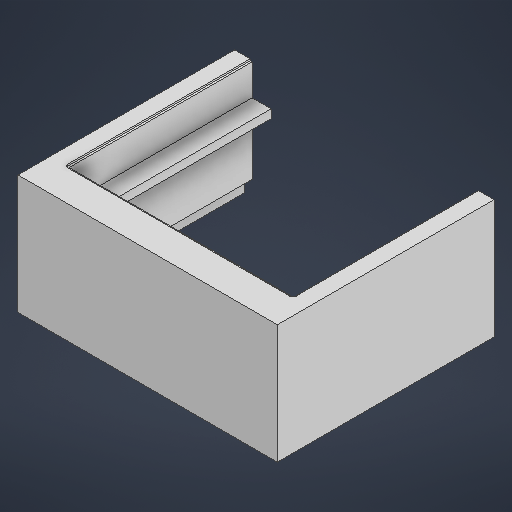
# Autodesk Inventor part: Enclosure
Saved by Autodesk Inventor 2025.2 (Build 292293000, 293)
## iProperties
Created: 2025-02-10
Part Number: Enclosure
Material: Generic
Document SubType Name: Modeling
Designer: elier
Density: 1 g/cm^3
Appearance: Default
Author: elier
Autodesk Inventor part; units mm, degrees
ref_plane "YZ Plane" through (0, 0, 0) normal (1, 0, 0) x (0, 1, 0)
ref_plane "XZ Plane" through (0, 0, 0) normal (0, 1, 0) x (-1, 0, 0)
ref_plane "XY Plane" through (0, 0, 0) normal (0, 0, 1) x (1, 0, 0)
sketch "Sketch1" plane through (0, 0, 0) normal (0, 1, 0) x (-1, 0, 0)
  line L0 (-83.5, 139.5) -> (83.5, 139.5)
  line L1 (83.5, 139.5) -> (83.5, -139.5)
  line L2 (83.5, -139.5) -> (-83.5, -139.5)
  line L3 (-83.5, -139.5) -> (-83.5, 139.5)
  line L4 (-83.5, 139.5) -> (83.5, -139.5) construction
  line L5 (83.5, 139.5) -> (-83.5, -139.5) construction
  point P0 (0, 0)
  dimension "d0" = 167
  dimension "d1" = 279
  constraints: 12 end point, 2 midpoint, 2 parallel, 1 horizontal, 1 perpendicular
  measures "d0" distance of L1.end L2.end
  measures "d1" distance of L0.end L1.end
extrude "Extrusion1" add sketch "Sketch1" along normal blind 26.6
sketch "Sketch2" plane through (0, 26.6, 0) normal (0, 1, 0) x (1, 0, 0)
  line L0 (71.5, -119.5) -> (-71.5, -119.5)
  line L1 (-73.5, -117.5) -> (-73.5, 117.5)
  line L2 (-71.5, 119.5) -> (71.5, 119.5)
  line L3 (73.5, 117.5) -> (73.5, -117.5)
  line L4 (73.5, -119.5) -> (-73.5, 119.5) construction
  line L5 (-73.5, -119.5) -> (73.5, 119.5) construction
  arc A0 (-73.5, -117.5) -> (-71.5, -119.5) centre (-71.5, -117.5) ccw
  arc A1 (-71.5, 119.5) -> (-73.5, 117.5) centre (-71.5, 117.5) ccw
  arc A2 (73.5, 117.5) -> (71.5, 119.5) centre (71.5, 117.5) ccw
  arc A3 (71.5, -119.5) -> (73.5, -117.5) centre (71.5, -117.5) ccw
  point P0 (0, 0)
  dimension "d4" = 147
  dimension "d5" = 239
  dimension "d6" = 2
  constraints: 12 end point, 8 point on circle, 8 point on line, 8 tangent, 4 centre point, 3 equal radius, 2 midpoint, 2 parallel, 1 horizontal, 1 perpendicular
  measures "d4" distance of L4.end L5.end
  measures "d5" distance of L5.start L4.end
  measures "d6" radius of A0
extrude "Extrusion2" cut sketch "Sketch2" against normal blind 1.1
sketch "Sketch3" plane through (0, 25.5, 0) normal (0, 1, 0) x (1, 0, 0)
  line L0 (-73.5, -117.5) -> (-73.5, 117.5) projected
  line L1 (71.5, -119.5) -> (-71.5, -119.5) projected
  line L2 (-72.25, -117.83) -> (72.25, -117.83)
  line L3 (72.25, -117.83) -> (72.25, 112.27)
  line L4 (72.25, 112.27) -> (-72.25, 112.27)
  line L5 (-72.25, 112.27) -> (-72.25, -117.83)
  point P0 (0, 0)
  dimension "d9" = 1.25
  dimension "d10" = 1.67
  dimension "d11" = 144.5
  dimension "d12" = 230.1
  constraints: 8 end point, 2 parallel, 1 horizontal, 1 perpendicular
  measures "d9" distance from line of L0 L2.start
  measures "d10" distance from line of L1 L2.start
  measures "d11" distance of L4.end L3.end
  measures "d12" distance of L3.end L2.end
extrude "Extrusion3" cut sketch "Sketch3" against normal blind 20
sketch "Sketch4" plane through (0, 5.5, 0) normal (0, 1, 0) x (1, 0, 0)
  circle A0 centre (-66.5, -111.83) radius 2
  line L0 (72.25, -117.83) -> (-72.25, -117.83) projected
  line L1 (-72.25, -117.83) -> (-72.25, 112.27) projected
  circle A1 centre (66.5, -111.83) radius 2
  line L2 (72.25, 112.27) -> (72.25, -117.83) projected
  circle A2 centre (-66.5, 106.27) radius 2
  line L3 (-72.25, 112.27) -> (72.25, 112.27) projected
  circle A3 centre (66.5, 106.27) radius 2
  point P0 (0, 0)
  dimension "d15" = 4
  dimension "d16" = 6
  dimension "d17" = 5.75
  dimension "d18" = 4
  dimension "d19" = 6
  dimension "d20" = 5.75
  dimension "d21" = 4
  dimension "d22" = 5.75
  dimension "d23" = 6
  dimension "d24" = 4
  dimension "d25" = 6
  dimension "d26" = 5.75
  constraints: 4 centre point
  measures "d15" diameter of A0
  measures "d16" distance from line of L0 A0.centre
  measures "d17" distance from line of L1 A0.centre
  measures "d18" diameter of A1
  measures "d19" distance from line of L0 A1.centre
  measures "d20" distance from line of L2 A1.centre
  measures "d21" diameter of A2
  measures "d22" distance from line of L1 A2.centre
  measures "d23" distance from line of L3 A2.centre
  measures "d24" diameter of A3
  measures "d25" distance from line of L3 A3.centre
  measures "d26" distance from line of L2 A3.centre
extrude "Extrusion4" add sketch "Sketch4" along normal blind 10.3 contours A0 | A1 | A2 | A3
sketch "Sketch5" plane through (0, 5.5, 0) normal (0, 1, 0) x (1, 0, 0)
  circle A0 centre (-66.5, -111.83) radius 2 projected
  circle A1 centre (-66.5, -111.83) radius 1.25
  circle A2 centre (-66.5, 106.27) radius 2 projected
  circle A3 centre (-66.5, 106.27) radius 1.25
  circle A4 centre (66.5, 106.27) radius 2 projected
  circle A5 centre (66.5, 106.27) radius 1.25
  circle A6 centre (66.5, -111.83) radius 1.25
  point P0 (0, 0)
  dimension "d29" = 2.5
  dimension "d30" = 2.5
  dimension "d31" = 2.5
  dimension "d32" = 2.5
  constraints: 4 centre point, 3 coincident
  measures "d29" diameter of A1
  measures "d30" diameter of A3
  measures "d31" diameter of A5
  measures "d32" diameter of A6
extrude "Extrusion5" cut sketch "Sketch5" along normal blind 10.3 and the other way blind 5.5 contours A1 | A3 | A5 | A6
sketch "Sketch8" plane through (0, 0, 0) normal (0, -1, 0) x (1, 0, 0)
  circle A0 centre (66.5, 111.83) radius 1.25 projected
  circle A1 centre (66.5, 111.83) radius 1.75
  circle A2 centre (66.5, -106.27) radius 1.25 projected
  circle A3 centre (66.5, -106.27) radius 1.75
  circle A4 centre (-66.5, -106.27) radius 1.25 projected
  circle A5 centre (-66.5, -106.27) radius 1.75
  circle A6 centre (-66.5, 111.83) radius 1.75
  point P0 (0, 0)
  dimension "d49" = 3.5
  dimension "d50" = 3.5
  dimension "d51" = 3.5
  dimension "d52" = 3.5
  constraints: 4 centre point, 3 coincident
  measures "d49" diameter of A1
  measures "d50" diameter of A3
  measures "d51" diameter of A5
  measures "d52" diameter of A6
extrude "Extrusion8" cut sketch "Sketch8" against normal blind 13.8
sketch "Sketch9" plane through (0, 5.5, 0) normal (0, 1, 0) x (1, 0, 0)
  line L0 (60, -100) -> (-60, -100)
  line L1 (-60, -100) -> (-60, 100)
  line L2 (-60, 100) -> (60, 100)
  line L3 (60, 100) -> (60, -100)
  line L4 (60, -100) -> (-60, 100) construction
  line L5 (-60, -100) -> (60, 100) construction
  point P0 (0, 0)
  dimension "d55" = 120
  dimension "d56" = 200
  constraints: 12 end point, 2 midpoint, 2 parallel, 1 horizontal, 1 perpendicular
  measures "d55" distance of L1.end L2.end
  measures "d56" distance of L0.end L1.end
extrude "Extrusion9" cut sketch "Sketch9" against normal blind 5.8
sketch "Sketch10" plane through (0, 0, 0) normal (0, -1, 0) x (1, 0, 0)
  line L0 (83.5, 139.5) -> (83.5, -139.5) projected
  line L1 (-83.5, -139.5) -> (-83.5, 139.5) projected
  line L2 (83.5, 139.5) -> (-83.5, 139.5)
  line L3 (-83.5, 139.5) -> (-83.5, -139.5)
  line L4 (-83.5, -139.5) -> (83.5, -139.5)
  line L5 (83.5, -139.5) -> (83.5, 139.5)
  line L6 (72.25, -115.05) -> (-72.25, -115.05)
  line L7 (-72.25, -115.05) -> (-72.25, 115.05)
  line L8 (-72.25, 115.05) -> (72.25, 115.05)
  line L9 (72.25, 115.05) -> (72.25, -115.05)
  line L10 (72.25, -115.05) -> (-72.25, 115.05) construction
  line L11 (-72.25, -115.05) -> (72.25, 115.05) construction
  line L12 (-83.5, -139.5) -> (83.5, -139.5)
  line L13 (83.5, -139.5) -> (83.5, 139.5)
  line L14 (83.5, 139.5) -> (-83.5, 139.5)
  line L15 (-83.5, 139.5) -> (-83.5, -139.5)
  point P0 (0, 0)
  point P1 (71.5, 119.5)
  dimension "d67" = 144.5
  dimension "d68" = 230.1
  constraints: 28 end point, 6 parallel, 3 horizontal, 3 perpendicular, 2 midpoint
  measures "d67" distance of L7.end L8.end
  measures "d68" distance of L6.end L7.end
extrude "Extrusion10" add sketch "Sketch10" along normal blind 40
sketch "Sketch12" plane through (0, -40, 0) normal (0, -1, 0) x (1, 0, 0)
  line L0 (-72.25, -115.05) -> (-72.25, 115.05) projected
  line L1 (72.25, -115.05) -> (-72.25, -115.05) projected
  line L2 (-77.25, -120.05) -> (-72.25, -120.05)
  line L3 (-72.25, -120.05) -> (-72.25, 120.05)
  line L4 (-72.25, 120.05) -> (-77.25, 120.05)
  line L5 (-77.25, 120.05) -> (-77.25, -120.05)
  line L6 (72.25, 115.05) -> (72.25, -115.05) projected
  line L7 (77.25, -120.05) -> (72.25, -120.05)
  line L8 (72.25, -120.05) -> (72.25, 120.05)
  line L9 (72.25, 120.05) -> (77.25, 120.05)
  line L10 (77.25, 120.05) -> (77.25, -120.05)
  line L11 (72.25, 115.05) -> (-72.25, 115.05) projected
  line L12 (72.25, 120.05) -> (-72.25, 120.05)
  line L13 (-72.25, 120.05) -> (-72.25, 115.05)
  line L14 (-72.25, 115.05) -> (72.25, 115.05)
  line L15 (72.25, 115.05) -> (72.25, 120.05)
  line L16 (-83.5, 139.5) -> (-83.5, -139.5) projected
  line L17 (83.5, 139.5) -> (-83.5, 139.5) projected
  line L18 (-83.5, -139.5) -> (83.5, -139.5)
  line L19 (83.5, -139.5) -> (83.5, 139.5)
  line L20 (83.5, 139.5) -> (-83.5, 139.5)
  line L21 (-83.5, 139.5) -> (-83.5, -139.5)
  line L22 (-72.25, -115.05) -> (72.25, -115.05) projected
  line L23 (-72.25, -115.05) -> (72.25, -115.05)
  line L24 (72.25, -115.05) -> (72.25, -120.05)
  line L25 (72.25, -120.05) -> (-72.25, -120.05)
  line L26 (-72.25, -120.05) -> (-72.25, -115.05)
  point P0 (0, 0)
  dimension "d69" = 5
  dimension "d70" = 5
  dimension "d71" = 240.1
  dimension "d72" = 5
  dimension "d73" = 5
  dimension "d74" = 240.1
  constraints: 40 end point, 10 parallel, 5 horizontal, 5 perpendicular, 1 point on line
  measures "d69" distance from line of L2.start L0
  measures "d70" distance from line of L1 L2.start
  measures "d71" distance of L3.end L2.end
  measures "d72" distance from line of L7.start L1
  measures "d73" distance from line of L6 L7.start
  measures "d74" distance of L7.end L8.end
extrude "Extrusion11" add sketch "Sketch12" along normal blind 10
sketch "Sketch13" plane through (0, -50, 0) normal (0, -1, 0) x (1, 0, 0)
  circle A0 centre (-77.5, -133.5) radius 1.25
  line L0 (-83.5, 139.5) -> (-83.5, -139.5) projected
  line L1 (-83.5, -139.5) -> (83.5, -139.5) projected
  circle A1 centre (-77.5, 133.5) radius 1.25
  line L2 (83.5, 139.5) -> (-83.5, 139.5) projected
  circle A2 centre (77.5, 133.5) radius 1.25
  line L3 (83.5, -139.5) -> (83.5, 139.5) projected
  circle A3 centre (77.5, -133.5) radius 1.25
  point P0 (0, 0)
  dimension "d77" = 2.5
  dimension "d78" = 6
  dimension "d79" = 6
  dimension "d80" = 2.5
  dimension "d81" = 6
  dimension "d82" = 6
  dimension "d83" = 2.5
  dimension "d84" = 6
  dimension "d85" = 6
  dimension "d86" = 6
  dimension "d87" = 6
  constraints: 4 centre point
  measures "d77" diameter of A0
  measures "d78" distance from line of L0 A0.centre
  measures "d79" distance from line of L1 A0.centre
  measures "d80" diameter of A1
  measures "d81" distance from line of L0 A1.centre
  measures "d82" distance from line of L2 A1.centre
  measures "d83" diameter of A2
  measures "d84" distance from line of L2 A2.centre
  measures "d85" distance from line of L3 A2.centre
  measures "d86" distance from line of L1 A3.centre
  measures "d87" distance from line of L3 A3.centre
extrude "Extrusion12" cut sketch "Sketch13" against normal blind 10 contours A0 | A1 | A2 | A3
sketch "Sketch14" plane through (83.5, 26.6, 139.5) normal (1, 0, 0) x (0, 0, -1)
  line L0 (0, 0) -> (279, 0) projected
  line L1 (139.5, 0) -> (139.5, -76.6)
  line L2 (259.55, -76.6) -> (19.45, -76.6) projected
  point P0 (139.5, -26.6)
  constraints: 2 end point, 2 midpoint
split_face "Split1"
sketch "Sketch18" plane through (83.5, -50, 0) normal (1, 0, 0) x (0, 0, -1)
  line L0 (0, 76.6) -> (139.5, 76.6) projected
  line L1 (139.5, 76.6) -> (139.5, 0) projected
  line L2 (0, 76.6) -> (139.5, 76.6)
  line L3 (139.5, 76.6) -> (139.5, 0)
  line L4 (139.5, 0) -> (0, 0)
  line L5 (0, 0) -> (0, 76.6)
  point P0 (0, 50)
  constraints: 8 end point, 2 parallel, 1 horizontal, 1 perpendicular
extrude "Extrusion15" cut sketch "Sketch18" against normal blind 168.1125
sketch "Sketch19" plane through (83.5, -50, 0) normal (0, 0, -1) x (-1, 0, 0)
  line L0 (0, 76.6) -> (10, 76.6) projected
  circle A0 centre (5, 66) radius 2.5
  circle A1 centre (5, 46) radius 2.5
  circle A2 centre (5, 26) radius 2.5
  line L1 (157, 76.6) -> (167, 76.6) projected
  circle A3 centre (162, 66) radius 2.5
  circle A4 centre (162, 46) radius 2.5
  circle A5 centre (162, 26) radius 2.5
  point P0 (83.5, 50)
  dimension "d97" = 5
  dimension "d99" = 5
  dimension "d101" = 5
  dimension "d102" = 5
  dimension "d104" = 5
  dimension "d106" = 5
  constraints: 6 centre point
  measures "d97" diameter of A0
  measures "d99" diameter of A1
  measures "d101" diameter of A2
  measures "d102" diameter of A3
  measures "d104" diameter of A4
  measures "d106" diameter of A5
extrude "Extrusion16" cut sketch "Sketch19" against normal blind 15
body "Solid1"
